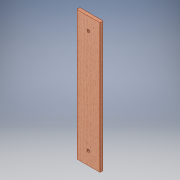
# Autodesk Inventor part: doga_short
Saved by Autodesk Inventor 2019 (Build 230136000, 136)
## iProperties
Created: 2019-02-23
Part Number: doga_short
Material: Wood (Oak)
Document SubType Name: Modeling
Designer: gaincarlo
Density: 0.76 g/cm^3
Appearance: White Oak - Natural Medium Gloss
Mass: 407.663 g
Surface Area: 1028.76 cm^2
Volume: 536.398 cm^3
Author: gaincarlo
Autodesk Inventor part; units mm, degrees
ref_plane "YZ Plane" through (0, 0, 0) normal (1, 0, 0) x (0, 1, 0)
ref_plane "XZ Plane" through (0, 0, 0) normal (0, 1, 0) x (-1, 0, 0)
ref_plane "Work Plane1" through (0, 0, 0) normal (0, 0, 1) x (1, 0, 0)
sketch "Sketch1" plane through (0, 0, 0) normal (0, 0, 1) x (1, 0, 0)
  line L0 (-45, -250) -> (45, -250)
  line L1 (45, -250) -> (45, 250)
  line L2 (45, 250) -> (-45, 250)
  line L3 (-45, 250) -> (-45, -250)
  line L4 (0, -250) -> (0, 250) construction
  circle A0 centre (0, -200) radius 5
  line L5 (-45, 0) -> (126, 0) construction
  circle A1 centre (0, 200) radius 5
  dimension "d0" = 90
  dimension "d1" = 500
  dimension "d10" = 10
  dimension "d11" = 200
  constraints: 12 end point, 3 midpoint, 2 centre point, 2 horizontal, 2 parallel, 1 perpendicular, 1 point on line, 1 symmetric about line, 1 other
  measures "d0" distance of L2.end L1.end
  measures "d1" distance of L1.end L0.end
  measures "d10" diameter of A0
  measures "d11" distance from line of A0.centre L5
extrude "Extrusion1" add sketch "Sketch1" along normal blind 12
fillet "Fillet1" radius 2 4 edges at (-45, 0, 12) (-45, 0, 0) (45, 0, 12) (45, 0, 0)
body "Solid1"
